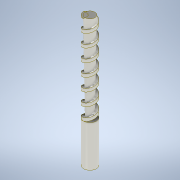
# Autodesk Inventor part: Husillo 8mm
Saved by Autodesk Inventor 2021 (Build 250183000, 183)
## iProperties
Created: 2021-10-26
Part Number: Husillo 8mm
Material: Acero
Document SubType Name: Modeling
Designer: arman
Density: 7.85 g/cm^3
Appearance: Plata
D_husillo_conex: 8,000 mm
Author: arman
Autodesk Inventor part; units mm, degrees
ref_plane "YZ Plane" through (0, 0, 0) normal (1, 0, 0) x (0, 1, 0)
sketch "Boceto1" plane through (0, 0, 0) normal (0, 1, 0) x (-1, 0, 0)
  circle A0 centre (0, 0) radius 4
  dimension "D_husillo_conex" = 8
  constraints: 1 centre point, 1 coincident
  measures "D_husillo_conex" diameter of A0
extrude "Ex_conexión" add sketch "Boceto1" along normal blind 26
sketch "B_dia_alma_inicio" plane through (0, 26, 0) normal (0, 1, 0) x (1, 0, 0)
  circle A0 centre (0, 0) radius 2.25
  dimension "D_alma_inic" = 4.5
  constraints: 1 centre point, 1 coincident
  measures "D_alma_inic" diameter of A0
ref_plane "Plano final husillo" through (0, 82, 0) normal (0, -1, 0) x (1, 0, 0)
sketch "Boceto3" plane through (0, 82, 0) normal (0, -1, 0) x (1, 0, 0)
  circle A0 centre (0, 0) radius 3.1
  dimension "D_alma_final" = 6.2
  constraints: 1 centre point, 1 coincident
  measures "D_alma_final" diameter of A0
loft "Ex_alma" add profiles "B_dia_alma_inicio", "Boceto3" separate body
sketch "B_filete" plane through (0, 0, 0) normal (0, 0, 1) x (1, 0, 0)
  line L0 (4, 26) -> (-4, 26) projected
  line L1 (-4, 24) -> (-4, 26)
  line L2 (0, 0) -> (0, 88.3214) construction
  line L3 (-4, 26) -> (-1, 26)
  line L4 (-4, 24) -> (-1, 24)
  line L5 (-1, 24) -> (-1, 26)
  dimension "Ancho_filete" = 0
  dimension "Alto_filete" = 3
  constraints: 10 end point, 2 perpendicular, 2 vertical
  measures "Ancho_filete" distance of L0.end L1.end
  measures "Alto_filete" distance of L1.end L3.end
coil "Bobina1" sketch "B_filete" operation add axis through (0, 0, 0) along (0, 1, 0) pitch 8 turns 7.5 hand right separate body
sketch "Boceto5" plane through (0, 82, 0) normal (0, 1, 0) x (1, 0, 0)
  circle A0 centre (0, 0) radius 5.7559
  constraints: 1 centre point, 1 coincident
extrude "Ex_corte" cut sketch "Boceto5" along normal blind 4.25 bodies 2 3
ref_plane "Plano de trabajo2" through (0, 10, 0) normal (0, -1, 0) x (1, 0, 0)
sketch "Boceto6" plane through (0, 10, 0) normal (0, -1, 0) x (1, 0, 0)
  circle A0 centre (0, 0) radius 4 projected
  circle A1 centre (0, 0) radius 4.075
  circle A2 centre (0, 0) radius 7.075
  dimension "d23" = 8.15
  dimension "d24" = 3
  constraints: 2 centre point, 1 coincident
  measures "d23" diameter of A1
  measures "d24" radial gap between concentric circles of A1 A2
extrude "Extrusión3" [suppressed]
ref_plane "Plano de trabajo3" through (0, 32, 0) normal (0, 1, 0) x (1, 0, 0)
sketch "Boceto7" plane through (0, 32, 0) normal (0, 1, 0) x (1, 0, 0)
  line L0 (-3.6945, -3.0475) -> (-8.2749, -6.8258)
  line L1 (-4.649, -1.8904) -> (-9.2294, -5.6686)
  line L2 (-2.74, -4.2047) -> (-7.3204, -7.9829)
  line L3 (-9.2294, -5.6686) -> (-7.3204, -7.9829)
  line L4 (-0.9545, 1.1571) -> (0.9545, -1.1571)
  line L5 (3.6945, 3.0475) -> (8.2749, 6.8258)
  line L6 (2.74, 4.2047) -> (7.3204, 7.9829)
  line L7 (4.649, 1.8904) -> (9.2294, 5.6686)
  line L8 (7.3204, 7.9829) -> (9.2294, 5.6686)
  line L9 (-2.74, -4.2047) -> (-4.649, -1.8904)
  line L10 (4.649, 1.8904) -> (2.74, 4.2047)
  point P0 (0, 0)
  dimension "d28" = 1.5
  dimension "d29" = 1.5
  constraints: 22 end point, 5 symmetric about line, 2 midpoint, 2 parallel, 1 perpendicular
  measures "d28" distance between parallel lines of L0 L1
  measures "d29" distance between parallel lines of L0 L2
ref_plane "Plano de trabajo4" through (0, 17, 0) normal (0, 1, 0) x (1, 0, 0)
sketch "Boceto8" plane through (0, 17, 0) normal (0, 1, 0) x (1, 0, 0)
  line L0 (-6.7703, 8.4544) -> (-8.8298, 6.2729)
  line L1 (8.8298, -6.2729) -> (6.7703, -8.4544)
  line L2 (-4.1148, 1.8217) -> (-8.8298, 6.2729)
  line L3 (-3.2722, 3.0891) -> (-7.8001, 7.3637)
  line L4 (-2.0554, 4.0032) -> (-6.7703, 8.4544)
  line L5 (4.1148, -1.8217) -> (8.8298, -6.2729)
  line L6 (3.2722, -3.0891) -> (7.8001, -7.3637)
  line L7 (2.0554, -4.0032) -> (6.7703, -8.4544)
  arc A0 (2.0554, -4.0032) -> (4.1148, -1.8217) centre (0, 0) ccw
  arc A1 (-2.0554, 4.0032) -> (-4.1148, 1.8217) centre (0, 0) ccw
  constraints: 16 end point, 6 point on circle, 2 centre point
equation "\"d14\" = Numero_filete_husillo"
equation "\"Numero_filete_husillo\" = 7.5"
